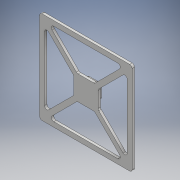
# Autodesk Inventor part: Base
Saved by Autodesk Inventor 2018 (Build 220112000, 112)
## iProperties
Created: 2018-03-07
Part Number: Base
Material: Generic
Document SubType Name: Modeling
Designer: sterl
Density: 1 g/cm^3
Appearance: Default
Author: sterl
Autodesk Inventor part; units mm, degrees
ref_plane "YZ Plane" through (0, 0, 0) normal (1, 0, 0) x (0, 1, 0)
ref_plane "XZ Plane" through (0, 0, 0) normal (0, 1, 0) x (-1, 0, 0)
ref_plane "XY Plane" through (0, 0, 0) normal (0, 0, 1) x (1, 0, 0)
sketch "Sketch1" plane through (0, 0, 0) normal (0, 1, 0) x (-1, 0, 0)
  line L0 (-95, 95) -> (95, 95)
  line L1 (95, 95) -> (95, -95)
  line L2 (95, -95) -> (-95, -95)
  line L3 (-95, -95) -> (-95, 95)
  line L4 (-95, 95) -> (95, -95) construction
  line L5 (95, 95) -> (-95, -95) construction
  point P0 (0, 0)
  dimension "d0" = 190
  dimension "d1" = 190
  constraints: 12 end point, 2 midpoint, 2 parallel, 1 horizontal, 1 perpendicular
  measures "d0" distance of L1.end L2.end
  measures "d1" distance of L0.end L1.end
extrude "Extrusion1" add sketch "Sketch1" along normal blind 5
sketch "Sketch2" plane through (0, 5, 0) normal (0, 1, 0) x (1, 0, 0)
  line L0 (-15, -15) -> (15, -15)
  line L1 (15, -15) -> (15, 15)
  line L2 (15, 15) -> (-15, 15)
  line L3 (-15, 15) -> (-15, -15)
  line L4 (-15, -15) -> (15, 15) construction
  line L5 (15, -15) -> (-15, 15) construction
  point P0 (0, 0)
  dimension "d4" = 30
  dimension "d5" = 30
  constraints: 12 end point, 2 midpoint, 2 parallel, 1 horizontal, 1 perpendicular
  measures "d4" distance of L2.end L1.end
  measures "d5" distance of L1.end L0.end
extrude "Extrusion2" add sketch "Sketch2" along normal blind 12
sketch "Sketch3" plane through (0, 17, 0) normal (0, 1, 0) x (1, 0, 0)
  line L0 (-10, -2.5) -> (-4.3301, -2.5)
  line L1 (10, -2.5) -> (10, 2.5)
  line L2 (10, 2.5) -> (4.3301, 2.5)
  line L3 (-10, 2.5) -> (-10, -2.5)
  line L4 (-10, -2.5) -> (10, 2.5) construction
  line L5 (10, -2.5) -> (-10, 2.5) construction
  arc A0 (-4.3301, -2.5) -> (4.3301, -2.5) centre (0, 0) ccw
  arc A1 (4.3301, 2.5) -> (-4.3301, 2.5) centre (0, 0) ccw
  line L6 (4.3301, -2.5) -> (10, -2.5)
  line L7 (-4.3301, 2.5) -> (-10, 2.5)
  dimension "d9" = 20
  dimension "d10" = 5
  constraints: 16 end point, 5 parallel, 4 point on circle, 2 centre point, 2 horizontal, 2 midpoint, 2 perpendicular, 1 coincident, 1 point on line
  measures "d9" distance of L3.start L1.end
  measures "d10" distance of L1.end L1.start
extrude "Extrusion3" cut sketch "Sketch3" against normal blind 11
fillet "Fillet1" radius 5 4 edges at (-95, 2.5, 95) (-95, 2.5, -95) (95, 2.5, 95) (95, 2.5, -95)
fillet "Fillet2" radius 5 4 edges at (-15, 11, 15) (15, 11, 15) (15, 11, -15) (-15, 11, -15)
sketch "Sketch5" plane through (0, 5, 0) normal (0, 1, 0) x (1, 0, 0)
  line L0 (-15, -10) -> (-15, 10) projected
  arc A0 (-10, 15) -> (-15, 10) centre (-10, 10) ccw projected
  line L1 (-10, 15) -> (10, 15) projected
  arc A1 (15, 10) -> (10, 15) centre (10, 10) ccw projected
  line L2 (15, 10) -> (15, -10) projected
  arc A2 (10, -15) -> (15, -10) centre (10, -10) ccw projected
  line L3 (10, -15) -> (-10, -15) projected
  arc A3 (-15, -10) -> (-10, -15) centre (-10, -10) ccw projected
  arc A4 (95, 90) -> (90, 95) centre (90, 90) ccw projected
  line L4 (90, 95) -> (-90, 95) projected
  arc A5 (-90, 95) -> (-95, 90) centre (-90, 90) ccw projected
  line L5 (-95, 90) -> (-95, -90) projected
  arc A6 (-95, -90) -> (-90, -95) centre (-90, -90) ccw projected
  line L6 (-90, -95) -> (90, -95) projected
  arc A7 (90, -95) -> (95, -90) centre (90, -90) ccw projected
  line L7 (95, -90) -> (95, 90) projected
  arc A8 (15, 10) -> (10, 15) centre (10, 10) ccw projected
  line L8 (38.9645, 46.0355) -> (17.9289, 25)
  line L9 (38.9645, 46.0355) -> (77.9289, 85)
  line L10 (-38.9645, 46.0355) -> (-17.9289, 25)
  line L11 (-38.9645, 46.0355) -> (-77.9289, 85)
  line L12 (-77.9289, 85) -> (77.9289, 85)
  line L13 (17.9289, 25) -> (-17.9289, 25)
  line L14 (-4.3301, -2.5) -> (-10, -2.5) projected
  arc A9 (-4.3301, -2.5) -> (4.3301, -2.5) centre (0, 0) ccw projected
  line L15 (10, -2.5) -> (4.3301, -2.5) projected
  line L16 (10, 2.5) -> (10, -2.5) projected
  line L17 (4.3301, 2.5) -> (10, 2.5) projected
  arc A10 (4.3301, 2.5) -> (-4.3301, 2.5) centre (0, 0) ccw projected
  line L18 (-10, 2.5) -> (-4.3301, 2.5) projected
  line L19 (-10, -2.5) -> (-10, 2.5) projected
  line L20 (-4.3301, -2.5) -> (-10, -2.5) projected
  arc A11 (-4.3301, -2.5) -> (4.3301, -2.5) centre (0, 0) ccw projected
  line L21 (10, -2.5) -> (4.3301, -2.5) projected
  line L22 (10, 2.5) -> (10, -2.5) projected
  line L23 (4.3301, 2.5) -> (10, 2.5) projected
  arc A12 (4.3301, 2.5) -> (-4.3301, 2.5) centre (0, 0) ccw projected
  line L24 (-10, 2.5) -> (-4.3301, 2.5) projected
  line L25 (-10, -2.5) -> (-10, 2.5) projected
  arc A13 (4.3301, 2.5) -> (-4.3301, 2.5) centre (0, 0) ccw projected
  arc A14 (-4.3301, -2.5) -> (4.3301, -2.5) centre (0, 0) ccw projected
  line L26 (25, -17.9289) -> (25, 17.9289)
  line L27 (85, 77.9289) -> (85, -77.9289)
  line L28 (46.0355, -38.9645) -> (25, -17.9289)
  line L29 (46.0355, -38.9645) -> (85, -77.9289)
  line L30 (46.0355, 38.9645) -> (85, 77.9289)
  line L31 (46.0355, 38.9645) -> (25, 17.9289)
  line L32 (-17.9289, -25) -> (17.9289, -25)
  line L33 (77.9289, -85) -> (-77.9289, -85)
  line L34 (-38.9645, -46.0355) -> (-17.9289, -25)
  line L35 (-38.9645, -46.0355) -> (-77.9289, -85)
  line L36 (38.9645, -46.0355) -> (77.9289, -85)
  line L37 (38.9645, -46.0355) -> (17.9289, -25)
  line L38 (-25, 17.9289) -> (-25, -17.9289)
  line L39 (-85, -77.9289) -> (-85, 77.9289)
  line L40 (-46.0355, 38.9645) -> (-25, 17.9289)
  line L41 (-46.0355, 38.9645) -> (-85, 77.9289)
  line L42 (-46.0355, -38.9645) -> (-85, -77.9289)
  line L43 (-46.0355, -38.9645) -> (-25, -17.9289)
  dimension "d24" = 360
  constraints: 48 end point, 2 coincident, 1 horizontal, 1 parallel, 50 other
extrude "Extrusion4" cut sketch "Sketch5" against normal blind 32.75 contours L8 L13 L10 L11 L12 L9 | L26 L31 L30 L27 L29 L28 | L32 L37 L36 L33 L35 L34 | L38 L43 L42 L39 L41 L40
fillet "Fillet3" radius 5 16 edges at (85, 2.5, -77.9289) (77.9289, 2.5, -85) (-85, 2.5, -77.9289) (-77.9289, 2.5, -85) (-17.9289, 2.5, -25) (17.9289, 2.5, -25) (-25, 2.5, -17.9289) (-17.9289, 2.5, 25) (17.9289, 2.5, 25) (85, 2.5, 77.9289) (77.9289, 2.5, 85) (-77.9289, 2.5, 85) (-85, 2.5, 77.9289) (-25, 2.5, 17.9289) (25, 2.5, 17.9289) (25, 2.5, -17.9289)
body "Solid1"
